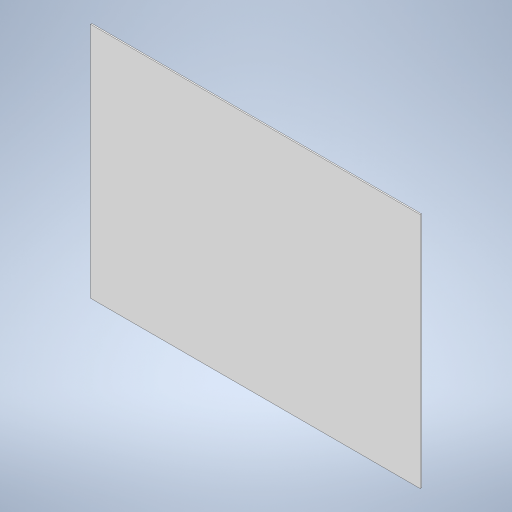
# Autodesk Inventor part: plate_side_with_logo
Saved by Autodesk Inventor 2023 (Build 270158000, 158)
## iProperties
Created: 2023-08-22
Part Number: plate_side_with_logo
Material: Polystyrene
Document SubType Name: Modeling
Designer: chriboehm
Density: 1.021 g/cm^3
Appearance: White
Mass: 1240.51 g
Surface Area: 8177.4 cm^2
Volume: 1215 cm^3
Author: chriboehm
Autodesk Inventor part; units mm, degrees
ref_plane "YZ Plane" through (0, 0, 0) normal (1, 0, 0) x (0, 1, 0)
ref_plane "XZ Plane" through (0, 0, 0) normal (0, 1, 0) x (-1, 0, 0)
ref_plane "XY Plane" through (0, 0, 0) normal (0, 0, 1) x (1, 0, 0)
sketch "Sketch1" plane through (0, 0, 0) normal (0, 0, 1) x (1, 0, 0)
  line L0 (-375, -270) -> (375, -270)
  line L1 (375, -270) -> (375, 270)
  line L2 (375, 270) -> (-375, 270)
  line L3 (-375, 270) -> (-375, -270)
  line L4 (-525, 0) -> (525, 0) projected
  line L5 (0, -378) -> (0, 378) projected
  dimension "d0" = 750
  dimension "d1" = 540
  constraints: 8 end point, 2 parallel, 1 horizontal, 1 perpendicular, 2 other
  measures "d0" distance of L1.end L2.end
  measures "d1" distance between parallel lines of L0 L2
extrude "Extrusion1" add sketch "Sketch1" along normal blind 3
ref_plane "Work Plane2" through (0, 0, 3) normal (0, 0, 1) x (1, 0, 0)
sketch "Sketch3" plane through (0, 0, 3) normal (0, 0, 1) x (1, 0, 0)
  line L0 (-375, 375) -> (375, 375) construction
  line L1 (375, 375) -> (375, -375) construction
  line L2 (375, -375) -> (-375, -375) construction
  line L3 (-375, -375) -> (-375, 375) construction
  line L4 (-375, 270) -> (-375, 0) projected
  line L5 (375, -270) -> (375, 270) projected
  line L6 (375, 270) -> (-375, 270) projected
  point P0 (0, 0)
  dimension "d28" = 0
  dimension "d29" = 750
  dimension "d30" = 750
  dimension "d35" = 540
  dimension "d38" = 750
  dimension "d39" = 105
  constraints: 2 other
  measures "d28" distance between parallel lines of L4 L3
  measures "d29" distance between parallel lines of L4 L5
  measures "d30" distance of L0.start L0.end
  measures "d35" distance of L5.start L5.end
  measures "d38" distance of L0.end L1.end
  measures "d39" distance between parallel lines of L6 L0
decal "Decal1"
equation "\"d28\" = -0.5 * d30 + 0.5 * d29"
equation "\"d30\" = d29"
equation "\"d39\" = -0.5 * d35 + 0.5 * d38"
body "Solid1"
